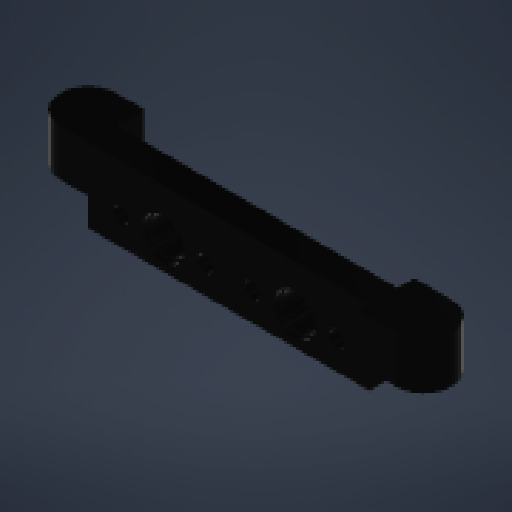
# Autodesk Inventor part: rmwall
Saved by Autodesk Inventor 2026.2 (Build 302298010, 298A)
## iProperties
Created: 2026-04-27
Part Number: rmwall
Material: Tworzywo sztuczne PET
Document SubType Name: Modeling
Designer: karol
Density: 1.541 g/cm^3
Appearance: Poliwęglan — przezroczysty
Author: karol
Autodesk Inventor part; units mm, degrees
ref_plane "YZ Plane" through (0, 0, 0) normal (1, 0, 0) x (0, 1, 0)
ref_plane "XZ Plane" through (0, 0, 0) normal (0, 1, 0) x (-1, 0, 0)
ref_plane "XY Plane" through (0, 0, 0) normal (0, 0, 1) x (1, 0, 0)
sketch "Szkic1" plane through (0, 0, 0) normal (0, 1, 0) x (-1, 0, 0)
  line L0 (0, 0) -> (42, 0)
  line L1 (42, 0) -> (42, -3)
  line L2 (42, -3) -> (0, -3)
  line L3 (0, -3) -> (0, 0)
  dimension "d0" = 42
  dimension "d1" = 3
  constraints: 8 end point, 2 parallel, 1 horizontal, 1 perpendicular
  measures "d0" distance of L1.end L2.end
  measures "d1" distance of L0.end L1.end
extrude "Wyciągnięcie proste1" add sketch "Szkic1" along normal blind 8
sketch "Szkic2" plane through (0, 8, 0) normal (0, 1, 0) x (1, 0, 0)
  circle A0 centre (-39.3616, 1.5) radius 1
  point P0 (0, 0)
  dimension "d4" = 2
  constraints: 1 centre point
  measures "d4" diameter of A0
extrude "Wyciągnięcie proste2" cut sketch "Szkic2" against normal blind 0.2
sketch "Szkic3" plane through (0, 0, -3) normal (0, 0, -1) x (-1, 0, 0)
  line L0 (0, 0) -> (42, 0) projected
  line L1 (0, 8) -> (42, 8) projected
  line L2 (42, 0) -> (36, 0)
  line L3 (36, 0) -> (36, 8)
  line L4 (36, 8) -> (42, 8)
  line L5 (42, 8) -> (42, 0)
  line L6 (0, 8) -> (6, 8)
  line L7 (6, 8) -> (6, 0)
  line L8 (6, 0) -> (0, 0)
  line L9 (0, 0) -> (0, 8)
  circle A0 centre (9.5, 3) radius 0.85
  circle A1 centre (18.5, 3) radius 0.85
  circle A2 centre (23.5, 3) radius 0.85
  circle A3 centre (32.5, 3) radius 0.85
  circle A4 centre (14, 3) radius 1.95
  circle A5 centre (28, 3) radius 1.95
  dimension "d7" = 6
  dimension "d8" = 6
  dimension "d9" = 1.7
  dimension "d10" = 1.7
  dimension "d11" = 1.7
  dimension "d12" = 1.7
  dimension "d13" = 3.5
  dimension "d14" = 3.5
  dimension "d15" = 3
  dimension "d16" = 3
  dimension "d17" = 3
  dimension "d18" = 3
  dimension "d19" = 9
  dimension "d20" = 9
  dimension "d21" = 3.9
  dimension "d22" = 3
  dimension "d23" = 4.5
  dimension "d24" = 3.9
  dimension "d25" = 3
  dimension "d26" = 4.5
  constraints: 16 end point, 6 centre point, 4 parallel, 2 horizontal, 2 perpendicular, 2 point on line
  measures "d7" distance of L3.end L4.end
  measures "d8" distance of L7.end L8.end
  measures "d9" diameter of A0
  measures "d10" diameter of A1
  measures "d11" diameter of A2
  measures "d12" diameter of A3
  measures "d13" distance from line of L3 A3.centre
  measures "d14" distance from line of L7 A0.centre
  measures "d15" distance from line of L0 A0.centre
  measures "d16" distance from line of L0 A1.centre
  measures "d17" distance from line of L0 A2.centre
  measures "d18" distance from line of L0 A3.centre
  measures "d19" distance of A1.centre A0.centre
  measures "d20" distance of A2.centre A3.centre
  measures "d21" diameter of A4
  measures "d22" distance from line of L0 A4.centre
  measures "d23" distance of A0.centre A4.centre
  measures "d24" diameter of A5
  measures "d25" distance from line of L0 A5.centre
  measures "d26" distance of A3.centre A5.centre
extrude "Wyciągnięcie proste3" cut sketch "Szkic3" against normal blind 3 contours A0 | A1 | A2 | A3 | A4 | A5
sketch "Szkic4" plane through (0, 8, 0) normal (0, 1, 0) x (1, 0, 0)
  line L0 (-42, 0) -> (0, 0) projected
  line L1 (-42, 0) -> (-36, 0)
  line L2 (-36, 0) -> (-36, 6)
  line L3 (-36, 6) -> (-42, 6)
  line L4 (-42, 6) -> (-42, 0)
  dimension "d29" = 6
  dimension "d30" = 6
  constraints: 8 end point, 2 parallel, 1 horizontal, 1 perpendicular
  measures "d29" distance of L3.end L2.end
  measures "d30" distance of L2.end L1.end
extrude "Wyciągnięcie proste4" add sketch "Szkic4" against normal blind 8
sketch "Szkic5" plane through (0, 0, 0) normal (0, -1, 0) x (1, 0, 0)
  line L0 (-42, 0) -> (0, 0) projected
  line L1 (-36, -3) -> (-36, -6) projected
  line L2 (-42, 0) -> (-36, 0)
  line L3 (-36, 0) -> (-36, -6)
  line L4 (-36, -6) -> (-42, -6)
  line L5 (-42, -6) -> (-42, 0)
  constraints: 8 end point, 2 parallel, 1 horizontal, 1 perpendicular
extrude "Wyciągnięcie proste5" cut sketch "Szkic5" against normal blind 3
sketch "Szkic20" plane through (0, 8, 0) normal (0, 1, 0) x (1, 0, 0)
  line L0 (0, 3) -> (-36, 3) projected
  line L1 (0, 0) -> (-6, 0)
  line L2 (-6, 0) -> (-6, 3)
  line L3 (-6, 3) -> (0, 3)
  line L4 (0, 3) -> (0, 0)
  line L5 (0, 0) -> (-6, 0)
  line L6 (-6, 0) -> (-6, 5.8)
  line L7 (-6, 5.8) -> (0, 5.8)
  line L8 (0, 5.8) -> (0, 0)
  line L9 (-6, 0) -> (2, 0)
  line L10 (2, 0) -> (2, -2.2)
  line L11 (2, -2.2) -> (-6, -2.2)
  line L12 (-6, -2.2) -> (-6, 0)
  line L13 (2, 0) -> (0, 0)
  line L14 (0, 0) -> (0, 5.8)
  line L15 (0, 5.8) -> (2, 5.8)
  line L16 (2, 5.8) -> (2, 0)
  dimension "d105" = 6
  dimension "d106" = 5.8
  dimension "d107" = 8
  dimension "d108" = 2.2
  constraints: 32 end point, 8 parallel, 4 horizontal, 4 perpendicular, 1 point on line
  measures "d105" distance of L2.end L3.end
  measures "d106" distance of L5.end L6.end
  measures "d107" distance of L10.end L11.end
  measures "d108" distance of L9.end L10.end
extrude "Wyciągnięcie proste23" add sketch "Szkic20" against normal blind 5
sketch "Szkic21" plane through (0, 0, 0) normal (0, -1, 0) x (1, 0, 0)
  line L0 (0, 0) -> (0, -3) projected
  line L1 (-6, 2.2) -> (-6, 0) projected
  line L2 (0, -3) -> (-6, -3)
  line L3 (-6, -3) -> (-6, 0)
  line L4 (-6, 0) -> (0, 0)
  line L5 (0, 0) -> (0, -3)
  constraints: 8 end point, 2 parallel, 1 horizontal, 1 perpendicular
extrude "Wyciągnięcie proste24" cut sketch "Szkic21" against normal blind 3
sketch "Szkic22" plane through (0, 3, 0) normal (0, -1, 0) x (1, 0, 0)
  circle A0 centre (-2, -1.8) radius 2
  line L0 (-6, -5.8) -> (2, -5.8) projected
  line L1 (2, -5.8) -> (2, 2.2) projected
  line L2 (-6, -3) -> (-6, -5.8) projected
  line L3 (-6, -5.8) -> (2, -5.8)
  line L4 (2, -5.8) -> (2, -4.8)
  line L5 (2, -4.8) -> (-6, -4.8)
  line L6 (-6, -4.8) -> (-6, -5.8)
  line L7 (2, -4.8) -> (1, -4.8)
  line L8 (1, -4.8) -> (1, 2.2)
  line L9 (1, 2.2) -> (2, 2.2)
  line L10 (2, 2.2) -> (2, -4.8)
  line L11 (1, 2.2) -> (-6, 2.2)
  line L12 (-6, 2.2) -> (-6, 1.2)
  line L13 (-6, 1.2) -> (1, 1.2)
  line L14 (1, 1.2) -> (1, 2.2)
  point P0 (0, 0)
  point P1 (-2, -5.8)
  point P2 (2, -1.8)
  point P3 (2, 2.2)
  point P4 (1, 1.2)
  dimension "d113" = 4
  dimension "d114" = 4
  dimension "d115" = 4
  dimension "d116" = 8
  dimension "d117" = 1
  dimension "d118" = 1
  dimension "d119" = 1
  constraints: 24 end point, 6 parallel, 3 horizontal, 3 perpendicular, 2 midpoint, 1 centre point, 1 point on line
  measures "d113" diameter of A0
  measures "d114" distance of point (-2, -5.8) A0.centre
  measures "d115" distance of point (2, -1.8) A0.centre
  measures "d116" distance of L5.end L4.end
  measures "d117" distance of L4.end L3.end
  measures "d118" distance of L8.end L9.end
  measures "d119" distance of L12.end L11.end
extrude "Wyciągnięcie proste25" cut sketch "Szkic22" against normal blind 3.25 contours A0
extrude "Wyciągnięcie proste26" cut sketch "Szkic22" against normal blind 5 contours L2 L5 L1 L0 | L5 L8 L9 L1 | L13 L12 L11 L8
sketch "Szkic25" plane through (-42, 3, 0) normal (0, 0, 1) x (1, 0, 0)
  circle A0 centre (28, 0) radius 1.95 projected
  circle A1 centre (28, 0) radius 2.2
  circle A2 centre (14, 0) radius 1.95 projected
  circle A3 centre (14, 0) radius 2.2
  point P0 (42, -3)
  dimension "d132" = 4.4
  dimension "d133" = 4.4
  constraints: 2 centre point, 2 coincident
  measures "d132" diameter of A1
  measures "d133" diameter of A3
extrude "Wyciągnięcie proste29" cut sketch "Szkic25" against normal blind 0.6 contours A0 | A1 | A2 | A3
sketch "Szkic26" plane through (0, 3, 0) normal (0, -1, 0) x (1, 0, 0)
  circle A0 centre (-39, -3) radius 2
  line L0 (-42, 0) -> (-36, 0) projected
  line L1 (-42, -6) -> (-42, 0) projected
  point P0 (0, 0)
  point P1 (-42, -3)
  dimension "d136" = 4
  dimension "d137" = 3
  dimension "d138" = 3
  constraints: 1 centre point, 1 midpoint
  measures "d136" diameter of A0
  measures "d137" distance from line of L0 A0.centre
  measures "d138" distance of point (-42, -3) A0.centre
extrude "Wyciągnięcie proste30" cut sketch "Szkic26" against normal blind 4
fillet "Fillet1" radius 3 4 edges at (-42, 5.5, -6) (1, 5.5, -4.8) (-42, 5.5, 0) (1, 5.5, 1.2)
chamfer "Chamfer1" distance 0.4 angle 45 4 edges at (-31.65, 3, -3) (-22.65, 3, -3) (-17.65, 3, -3) (-8.65, 3, -3)
